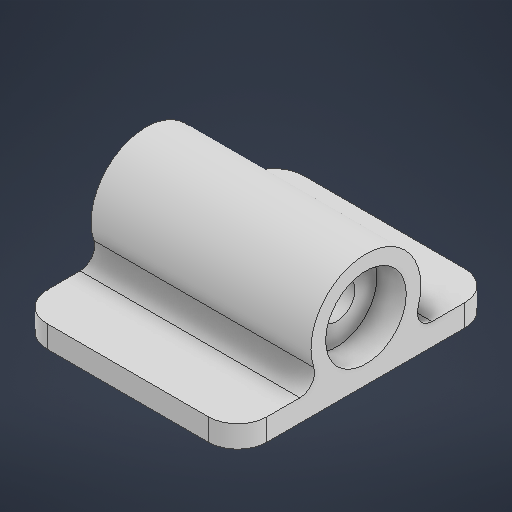
# Autodesk Inventor part: encaixeBase
Saved by Autodesk Inventor 2026.2 (Build 302298000, 298)
## iProperties
Created: 2026-02-13
Part Number: encaixeBase
Material: Genérico
Document SubType Name: Modeling
Designer: Ian
Density: 1 g/cm^3
Appearance: Padrão
Author: Ian
Autodesk Inventor part; units mm, degrees
ref_plane "YZ Plane" through (0, 0, 0) normal (1, 0, 0) x (0, 1, 0)
ref_plane "XZ Plane" through (0, 0, 0) normal (0, 1, 0) x (-1, 0, 0)
ref_plane "XY Plane" through (0, 0, 0) normal (0, 0, 1) x (1, 0, 0)
sketch "Esboço10" plane through (0, 0, 0) normal (1, 0, 0) x (0, 1, 0)
  line L0 (0, 0) -> (0, 17.5)
  line L1 (0, 0) -> (0, -17.5)
  line L2 (0, 17.5) -> (3, 17.5)
  circle A0 centre (8, 0) radius 2.5
  circle A1 centre (8, 0) radius 7.5
  line L3 (3, 17.5) -> (3, 5.5902)
  line L4 (0, -17.5) -> (3, -17.5)
  line L5 (3, -17.5) -> (3, -5.5902)
  dimension "d67" = 17.5
  dimension "d68" = 17.5
  dimension "d69" = 3
  dimension "d70" = 5
  dimension "d71" = 15
  dimension "d93" = 3
  dimension "d94" = 0
  dimension "d97" = 8
  constraints: 12 end point, 3 vertical, 2 centre point, 2 horizontal, 2 point on circle, 1 coincident, 1 perpendicular
  measures "d67" distance of L0.start L0.end
  measures "d68" distance of L0.start L1.end
  measures "d69" distance of L0.end L2.end
  measures "d70" diameter of A0
  measures "d71" diameter of A1
  measures "d93" distance of L1.end L4.end
  measures "d94" vertical distance of L0.start A0.centre
  measures "d97" distance from line of L1 A1.centre
extrude "Extrusão7" add sketch "Esboço10" along normal mid plane 30
fillet "Arredondamento5" radius 2 2 edges at (0, 3, 5.5902) (0, 3, -5.5902)
fillet "Arredondamento6" radius 4 4 edges at (15, 1.5, 17.5) (15, 1.5, -17.5) (-15, 1.5, 17.5) (-15, 1.5, -17.5)
sketch "Esboço15" plane through (15, 0, 0) normal (1, 0, 0) x (0, 0, -1)
  line L0 (13.5, 3) -> (13.5, 0) projected
  line L1 (13.5, 3) -> (9.0139, 3) projected
  arc A0 (7.1162, 5.6316) -> (9.0139, 3) centre (9.0139, 5) ccw projected
  arc A1 (7.1162, 5.6316) -> (-7.1162, 5.6316) centre (0, 8) ccw projected
  arc A2 (-9.0139, 3) -> (-7.1162, 5.6316) centre (-9.0139, 5) ccw projected
  line L2 (-9.0139, 3) -> (-13.5, 3) projected
  line L3 (-13.5, 0) -> (-13.5, 3) projected
  line L4 (-13.5, 0) -> (13.5, 0) projected
  circle A3 centre (0, 8) radius 2.5 projected
  circle A4 centre (0, 8) radius 5.5
  point P0 (0, 0)
  dimension "d98" = 11
  constraints: 1 centre point, 1 coincident
  measures "d98" diameter of A4
extrude "Extrusão11" cut sketch "Esboço15" against normal blind 4 contours A4
mirror "Espelhar1" about plane through (0, 0, 0) normal (1, 0, 0) of "Extrusão11"
equation "\"d68\" = d67"
